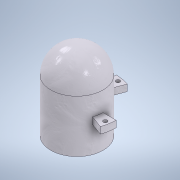
# Autodesk Inventor part: bottom tvc
Saved by Autodesk Inventor 2021 (Build 250183000, 183)
## iProperties
Created: 2021-07-19
Part Number: bottom tvc
Material: Aluminum 6061, Welded
Document SubType Name: Modeling
Designer: samlo
Density: 2.7 g/cm^3
Appearance: Weld - Aluminum
Author: samlo
Autodesk Inventor part; units mm, degrees
ref_plane "YZ Plane" through (0, 0, 0) normal (1, 0, 0) x (0, 1, 0)
ref_plane "XZ Plane" through (0, 0, 0) normal (0, 1, 0) x (-1, 0, 0)
ref_plane "XY Plane" through (0, 0, 0) normal (0, 0, 1) x (1, 0, 0)
sketch "Sketch1" plane through (0, 0, 0) normal (0, 0, 1) x (1, 0, 0)
  line L0 (20, 0) -> (20, 40)
  line L1 (0, 0) -> (0, 61)
  arc A0 (20, 40) -> (0, 60) centre (0, 40) ccw
  line L2 (19, 0) -> (19, 40)
  arc A1 (19, 40) -> (0, 59) centre (0, 40) ccw
  line L3 (19, 0) -> (20, 0)
  dimension "d0" = 40
  dimension "d1" = 20
  dimension "d21" = 19
  dimension "d22" = 38
  constraints: 8 end point, 4 point on circle, 3 point on line, 2 centre point, 2 vertical, 1 coincident, 1 horizontal, 1 parallel
  measures "d0" distance of L0.end L0.start
  measures "d1" distance from line of L0 L1.start
  measures "d21" distance of L2.start L1.start
  measures "d22" diameter of A1
revolve "Revolution1" add sketch "Sketch1" angle 360 about axis through (0, 0, 0) along (0, 1, 0)
sketch "Sketch2" plane through (0, 0, 0) normal (0, 0, 1) x (1, 0, 0)
  line L0 (20, 40) -> (20, 0) projected
  line L1 (20, 20) -> (30, 20)
  line L2 (30, 20) -> (30, 25)
  line L3 (30, 25) -> (20, 25)
  line L4 (-21, 0) -> (21, 0) projected
  line L5 (0, -8) -> (0, 48) projected
  point P0 (0, 0)
  dimension "d4" = 20
  dimension "d5" = 5
  dimension "d6" = 10
  constraints: 6 end point, 1 horizontal, 1 midpoint, 1 perpendicular, 1 point on line, 1 vertical, 1 other
  measures "d5" distance of L1.end L2.end
  measures "d6" distance of L1.start L1.end
revolve "Revolution2" add sketch "Sketch2" angle 20 about axis through (0, -10, 0) along (0, -1, 0)
sketch "Sketch3" plane through (21, 25, 0) normal (0, 1, 0) x (1, 0, 0)
  point P0 (-21, 0)
  point P1 (5.5271, -4.8663)
hole "Hole1" at (26.5271, 25, 4.8663) direction (0, -1, 0) diameter 3 end through all
pattern_circular "Circular Pattern1" count 2 over 90 about axis through (0, -10, 0) along (0, 1, 0) of "Revolution2"
pattern_circular "Circular Pattern2" count 2 over 90 about axis through (0, -10, 0) along (0, 1, 0) of "Hole1"
body "Solid1"
